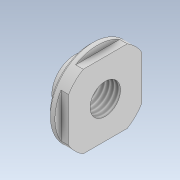
# Autodesk Inventor part: tuerca_manzana_1
Saved by Autodesk Inventor 2021 (Build 250183000, 183)
## iProperties
Created: 2021-04-24
Part Number: tuerca_manzana_1
Material: Genérico
Document SubType Name: Modeling
Designer: j2seb
Density: 1 g/cm^3
Appearance: Valor por defecto
Author: j2seb
Autodesk Inventor part; units mm, degrees
ref_plane "YZ Plane" through (0, 0, 0) normal (1, 0, 0) x (0, 1, 0)
ref_plane "XZ Plane" through (0, 0, 0) normal (0, 1, 0) x (-1, 0, 0)
ref_plane "XY Plane" through (0, 0, 0) normal (0, 0, 1) x (1, 0, 0)
sketch "Boceto1" plane through (0, 0, 0) normal (0, 0, 1) x (1, 0, 0)
  line L0 (0, 0) -> (11.3785, 0)
  line L1 (0, 5) -> (10, 5)
  line L2 (10, 5) -> (10, 14)
  line L3 (10, 14) -> (5, 14)
  line L4 (5, 14) -> (5, 7.5)
  line L5 (5, 7.5) -> (0, 7.5)
  line L6 (0, 7.5) -> (0, 5)
  dimension "d0" = 5
  dimension "d1" = 5
  dimension "d3" = 28
  dimension "d4" = 15
  dimension "d5" = 10
  constraints: 14 end point, 4 perpendicular, 3 horizontal, 1 vertical alignment
  measures "d0" distance of L4.end L5.end
  measures "d1" distance of L2.end L3.end
  measures "d3" diameter of L3 L0
  measures "d4" diameter of L5 L0
  measures "d5" diameter of L1 L0
revolve "Revolución1" add sketch "Boceto1" angle 360 about axis through (0, 0, 0) along (1, 0, 0)
fillet "Empalme1" radius 1 1 edges at (5, -7.5, 0)
chamfer "Chaflán1" distance 1 angle 45 1 edges at (5, -14, 0)
sketch "Boceto2" plane through (10, 0, 0) normal (1, 0, 0) x (0, 0, -1)
  circle A0 centre (0, 0) radius 14 projected
  line L0 (-12, 12) -> (12, 12)
  line L1 (12, 12) -> (12, -12)
  line L2 (12, -12) -> (-12, -12)
  line L3 (-12, -12) -> (-12, 12)
  point P0 (12, 0)
  point P1 (0, 12)
  point P2 (-7.2111, 12)
  point P3 (7.2111, 12)
  point P4 (12, 7.2111)
  point P5 (12, -7.2111)
  point P6 (-12, -7.2111)
  point P7 (-12, 7.2111)
  point P8 (7.2111, -12)
  point P9 (-7.2111, -12)
  dimension "d11" = 24
  dimension "d12" = 24
  constraints: 8 end point, 2 midpoint, 2 parallel, 1 horizontal, 1 horizontal alignment, 1 perpendicular, 1 vertical alignment
  measures "d11" distance of L0.end L1.end
  measures "d12" distance of L0.start L0.end
extrude "Extrusión1" cut sketch "Boceto2" against normal blind 2.5 contours A0 L1 | L0 A0 | A0 L2 | L3 A0
thread "Rosca1" size "M10x1.5" class "6H" standard "ANSI Metric M Profile" length 20
